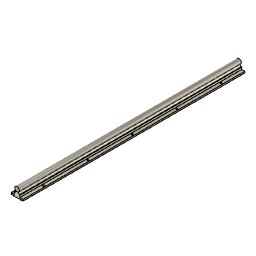
SBR16-750mm (Autodesk Fusion 360 design; units mm, degrees)
Autodesk Fusion 360 part; units mm, degrees
sketch "Alu Support" plane through (0, 0, 0) normal (0, 1, 0) x (1, 0, 0)
  line L0 (-20, 0.0005) -> (20, 0.0005)
  line L1 (20, 0.0005) -> (20, -4.9995)
  line L2 (20, -4.9995) -> (9.35, -4.9995)
  line L3 (9.35, -4.9995) -> (9.35, -11.6995)
  line L4 (9.35, -11.6995) -> (7.6, -11.6995)
  line L5 (7.6, -11.6995) -> (3.9691, -18.0536)
  line L6 (-3.9691, -18.0536) -> (-7.6, -11.6995)
  line L7 (-7.6, -11.6995) -> (-9.35, -11.6995)
  line L8 (-9.35, -11.6995) -> (-9.35, -4.9995)
  line L9 (-9.35, -4.9995) -> (-20, -4.9995)
  line L10 (-20, -4.9995) -> (-20, 0.0005)
  arc A0 (3.9691, -18.0536) -> (-3.9691, -18.0536) centre (0, -24.9995) ccw
  dimension "d3" = 40
  dimension "d4" = 18.7
  dimension "d5" = 1.75
  dimension "d6" = 25
  dimension "d7" = 6.7
  dimension "d8" = 5
  constraint horizontal L0
  constraint perpendicular L0 L1
  constraint perpendicular L1 L2
  constraint perpendicular L2 L3
  constraint perpendicular L1 L4
  constraint perpendicular L7 L8
  constraint perpendicular L8 L9
  constraint perpendicular L0 L10
  constraint equal L2 L9
  constraint equal L3 L8
  constraint equal L4 L7
  constraint equal L1 L10
  constraint parallel L0 L9
  measures "d3" distance of L1 L10
  measures "d4" distance of L3 L8
  measures "d5" distance of L6.end L7.end
  measures "d6" distance of L0 A0.centre
  measures "d7" distance of L2.end L3.end
  measures "d8" distance of L0 L9
sketch "Steel Rail" plane through (0, 0, 0) normal (0, 1, 0) x (1, 0, 0)
  circle A0 centre (0, -25) radius 8
extrude "Extrude1" add sketch "Alu Support" along normal mid plane 750 makes body 1
extrude "Extrude2" add sketch "Steel Rail" along normal mid plane 750 separate body makes body 2
copy_body "CutPasteBodies1" bodies 1 2 removing the originals makes body 3 makes body 4 in component "SBR16-750"
sketch "Holes" plane through (0, 0, -0.0005) normal (0, 0, -1) x (1, 0, 0)
  line L0 (-20, 375) -> (-20, -375)
  line L1 (-20, -375) -> (20, -375)
  line L2 (20, -375) -> (20, 375)
  line L3 (20, 375) -> (-20, 375)
  line L4 (15, 375) -> (15, -375) construction
  line L5 (-15, 375) -> (-15, -375) construction
  line L6 (25, 300) -> (-25, 300) construction
  line L7 (25, 150) -> (-25, 150) construction
  line L8 (25, 0) -> (-25, 0) construction
  line L9 (25, -150) -> (-25, -150) construction
  line L10 (25, -300) -> (-25, -300) construction
  circle A0 centre (15, -300) radius 2.75
  circle A1 centre (-15, -300) radius 2.75
  circle A2 centre (15, -150) radius 2.75
  circle A3 centre (-15, -150) radius 2.75
  circle A4 centre (-15, 0) radius 2.75
  circle A5 centre (15, 0) radius 2.75
  circle A6 centre (15, 150) radius 2.75
  circle A7 centre (-15, 150) radius 2.75
  circle A8 centre (15, 300) radius 2.75
  circle A9 centre (-15, 300) radius 2.75
  dimension "d15" = 5
  dimension "d16" = 5
  dimension "d17" = 30
  dimension "d18" = 150
  dimension "d19" = 150
  dimension "d20" = 150
  dimension "d21" = 150
  dimension "d22" = 75
  dimension "d23" = 75
  dimension "d24" = 5.5
  dimension "d25" = 5.5
  dimension "d26" = 5.5
  dimension "d27" = 5.5
  dimension "d28" = 5.5
  dimension "d29" = 5.5
  dimension "d30" = 5.5
  dimension "d31" = 5.5
  dimension "d32" = 5.5
  dimension "d33" = 5.5
  constraint coincident L3 L4.start
  constraint coincident L1 L4.end
  constraint perpendicular L1 L4
  constraint coincident L3 L5.start
  constraint coincident L1 L5.end
  constraint perpendicular L1 L5
  constraint perpendicular L0 L6
  constraint perpendicular L0 L7
  constraint perpendicular L0 L8
  constraint perpendicular L0 L9
  constraint perpendicular L0 L10
  constraint coincident L10 A0.centre
  constraint coincident L4 A0.centre
  constraint coincident L5 A1.centre
  constraint coincident L10 A1.centre
  constraint coincident L9 A2.centre
  constraint coincident L4 A2.centre
  constraint coincident L5 A3.centre
  constraint coincident L9 A3.centre
  constraint midpoint L5 A4.centre
  constraint midpoint L4 A5.centre
  constraint coincident L4 A6.centre
  constraint coincident L7 A6.centre
  constraint coincident L5 A7.centre
  constraint coincident L7 A7.centre
  constraint coincident L6 A8.centre
  constraint coincident L4 A8.centre
  constraint coincident L5 A9.centre
  constraint coincident L6 A9.centre
  measures "d15" distance of L2 L4
  measures "d16" distance of L0 L5
  measures "d17" distance of L4 L5
  measures "d18" distance of L9 L10
  measures "d19" distance of L8 L9
  measures "d20" distance of L7 L8
  measures "d21" distance of L6 L7
  measures "d22" distance of L2.end L6
  measures "d23" distance of L1 L10
  measures "d24" diameter of A0
  measures "d25" diameter of A1
  measures "d26" diameter of A2
  measures "d27" diameter of A3
  measures "d28" diameter of A4
  measures "d29" diameter of A5
  measures "d30" diameter of A6
  measures "d31" diameter of A7
  measures "d32" diameter of A8
  measures "d33" diameter of A9
extrude "Extrude1'" cut sketch "Holes" against normal blind 6 contours A8 | A9 bodies 3 in component "SBR16-750"
extrude "Extrude2'" cut sketch "Holes" against normal blind 6 contours A6 | A7 bodies 3 in component "SBR16-750"
extrude "Extrude3" cut sketch "Holes" against normal blind 6 contours A4 | A5 bodies 3 in component "SBR16-750"
extrude "Extrude4" cut sketch "Holes" against normal blind 6 contours A2 | A3 bodies 3 in component "SBR16-750"
extrude "Extrude5" cut sketch "Holes" against normal blind 6 contours A0 bodies 3 in component "SBR16-750"
extrude "Extrude6" cut sketch "Holes" against normal blind 6 contours A1 bodies 3 in component "SBR16-750"
component "SBR16-750" placed x (1, 0, 0) y (0, 1, 0) z (0, 0, 1) at (0, 0, 0)
named bodies: "Alu Support", "Steel Rail"
